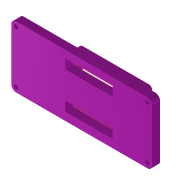
# Autodesk Inventor part: ESP32ParasiteMicroscope_base_v0
Saved by Autodesk Inventor 2022 (Build 260153000, 153)
## iProperties
Created: 2022-02-02
Part Number: ESP32ParasiteMicroscope_base_v0
Material: Generisch
Document SubType Name: Modeling
Designer: diederichbenedict
Density: 1 g/cm^3
Appearance: Glatt - Violett
Author: diederichbenedict
Autodesk Inventor part; units mm, degrees
ref_plane "YZ Plane" through (0, 0, 0) normal (1, 0, 0) x (0, 1, 0)
ref_plane "XZ Plane" through (0, 0, 0) normal (0, 1, 0) x (-1, 0, 0)
ref_plane "XY Plane" through (0, 0, 0) normal (0, 0, 1) x (1, 0, 0)
ref_plane "Arbeitsebene1" through (0, 0, 4) normal (0, 0, 1) x (1, 0, 0)
sketch "Skizze1" plane through (0, 0, 4) normal (0, 0, 1) x (1, 0, 0)
  arc A0 (-20, -12.5) -> (-19, -13.5) centre (-19, -12.5) ccw construction
  line L0 (-19, -13.5) -> (19, -13.5) construction
  arc A1 (19, -13.5) -> (20, -12.5) centre (19, -12.5) ccw construction
  line L1 (20, -12.5) -> (20, 12.5) construction
  arc A2 (20, 12.5) -> (19, 13.5) centre (19, 12.5) ccw construction
  line L2 (19, 13.5) -> (-19, 13.5) construction
  arc A3 (-19, 13.5) -> (-20, 12.5) centre (-19, 12.5) ccw construction
  line L3 (-20, 12.5) -> (-20, -12.5) construction
  line L4 (26, 12.5) -> (26, -12.5) construction
  arc A4 (19, -19.5) -> (26, -12.5) centre (19, -12.5) ccw construction
  line L5 (19, -19.5) -> (-19, -19.5) construction
  arc A5 (-26, -12.5) -> (-19, -19.5) centre (-19, -12.5) ccw construction
  line L6 (-26, -12.5) -> (-26, 12.5) construction
  arc A6 (-19, 19.5) -> (-26, 12.5) centre (-19, 12.5) ccw construction
  line L7 (-19, 19.5) -> (19, 19.5) construction
  arc A7 (26, 12.5) -> (19, 19.5) centre (19, 12.5) ccw construction
  line L8 (-24, 19.5) -> (19, 19.5)
  line L9 (19, 19.5) -> (19, -19.4749)
  line L10 (19, -19.4749) -> (-24, -19.4749)
  line L11 (-24, -19.4749) -> (-24, 19.5)
  line L12 (2.5735, 11.7657) -> (-15.3535, 11.7657) construction
  line L13 (2.5735, 13.7657) -> (-15.3535, 13.7657)
  line L14 (-15.3535, 9.7657) -> (2.5735, 9.7657)
  arc A8 (2.5735, 9.7657) -> (2.5735, 13.7657) centre (2.5735, 11.7657) ccw
  arc A9 (-15.3535, 13.7657) -> (-15.3535, 9.7657) centre (-15.3535, 11.7657) ccw
  line L15 (2.4395, -11.3613) -> (-15.3535, -11.3613) construction
  line L16 (2.4395, -9.3613) -> (-15.3535, -9.3613)
  line L17 (-15.3535, -13.3613) -> (2.4395, -13.3613)
  arc A10 (2.4395, -13.3613) -> (2.4395, -9.3613) centre (2.4395, -11.3613) ccw
  arc A11 (-15.3535, -9.3613) -> (-15.3535, -13.3613) centre (-15.3535, -11.3613) ccw
  circle A12 centre (-8.6034, 0.0126) radius 1.0539 construction
  line L18 (26.7026, 12.7126) -> (26.7026, -12.6874) construction
  line L19 (-48.7974, 12.7126) -> (26.7026, 12.7126) construction
  line L20 (-48.7974, -12.6874) -> (-48.7974, 12.7126) construction
  line L21 (26.7026, -12.6874) -> (-48.7974, -12.6874) construction
  line L22 (33.4901, -16.4749) -> (33.4901, 19.5) construction
  line L23 (30.4901, 19.5) -> (-52.5848, 19.5) construction
  line L24 (-55.5848, 19.5) -> (-55.5848, -16.4749) construction
  line L25 (-52.5848, -19.4749) -> (33.4901, -19.4749) construction
  line L26 (33.4901, 19.5) -> (19, 19.5)
  line L27 (19, 19.5) -> (19, -19.4749)
  line L28 (19, -19.4749) -> (30.4901, -19.4749)
  line L29 (33.4901, -19.4749) -> (33.4901, 16.5)
  line L30 (-24, 19.5) -> (-55.5848, 19.5)
  line L31 (-55.5848, 16.5) -> (-55.5848, -19.4749)
  line L32 (-55.5848, -19.4749) -> (-24, -19.4749)
  line L33 (-24, -19.4749) -> (-24, 19.5)
  arc A13 (-55.5848, -16.4749) -> (-52.5848, -19.4749) centre (-52.5848, -16.4749) ccw
  arc A14 (-52.5848, 19.5) -> (-55.5848, 16.5) centre (-52.5848, 16.5) ccw
  arc A15 (33.4901, 16.5) -> (30.4901, 19.5) centre (30.4901, 16.5) ccw
  arc A16 (30.4901, -19.4749) -> (33.4901, -16.4749) centre (30.4901, -16.4749) ccw
  line L34 (8.61, 8.7657) -> (-21.39, 8.7657)
  line L35 (-21.39, 8.7657) -> (-21.39, 14.7657)
  line L36 (-21.39, 14.7657) -> (8.61, 14.7657)
  line L37 (8.61, 14.7657) -> (8.61, 8.7657)
  line L38 (8.61, 8.7657) -> (-21.39, 14.7657) construction
  line L39 (-21.39, 8.7657) -> (8.61, 14.7657) construction
  line L40 (8.543, -14.3613) -> (-21.457, -14.3613)
  line L41 (-21.457, -14.3613) -> (-21.457, -8.3613)
  line L42 (-21.457, -8.3613) -> (8.543, -8.3613)
  line L43 (8.543, -8.3613) -> (8.543, -14.3613)
  line L44 (8.543, -14.3613) -> (-21.457, -8.3613) construction
  line L45 (-21.457, -14.3613) -> (8.543, -8.3613) construction
  point P0 (0, 0)
  point P1 (-15.2165, -11.3613)
  point P2 (-6.39, 11.7657)
  point P3 (-6.457, -11.3613)
  point P4 (-24, -18.4749)
  point P5 (33.4901, -16.4749)
  point P6 (30.4901, 19.5)
  point P7 (-52.5848, 19.5)
  point P8 (-55.5848, -16.4749)
  point P9 (-52.5848, -19.4749)
  dimension "d0" = 6
  dimension "d1" = 4
  dimension "d2" = 4
  dimension "d5" = 3
  dimension "d37" = 30
  dimension "d38" = 6
  dimension "d39" = 6
  dimension "d40" = 30
  constraints: 80 end point, 24 point on circle, 16 tangent, 15 parallel, 12 centre point, 9 point on line, 6 midpoint, 5 perpendicular, 4 horizontal, 3 equal radius, 14 other
  measures "d0" distance between parallel lines of L1 L4
  measures "d1" diameter of A9
  measures "d2" diameter of A11
  measures "d5" radius of A13
  measures "d37" distance of L34.start L34.end
  measures "d38" distance of L34.end L35.end
  measures "d39" distance of L40.end L41.end
  measures "d40" distance between parallel lines of L41 L43
extrude "Extrusion1" add sketch "Skizze1" along normal blind 5 contours L8 L9 L10 L11 | L11 L32 A13 L31 A14 L30 | L26 A15 L29 A16 L28 L9
sketch "Skizze3" plane through (0, 0, 4) normal (0, 0, -1) x (-1, 0, 0)
  arc A0 (-33.4901, -16.4749) -> (-30.4901, -19.4749) centre (-30.4901, -16.4749) ccw projected
  line L0 (52.5848, -19.4749) -> (-30.4901, -19.4749) projected
  arc A1 (52.5848, -19.4749) -> (55.5848, -16.4749) centre (52.5848, -16.4749) ccw projected
  line L1 (55.5848, 16.5) -> (55.5848, -16.4749) projected
  arc A2 (55.5848, 16.5) -> (52.5848, 19.5) centre (52.5848, 16.5) ccw projected
  line L2 (-30.4901, 19.5) -> (52.5848, 19.5) projected
  arc A3 (-30.4901, 19.5) -> (-33.4901, 16.5) centre (-30.4901, 16.5) ccw projected
  line L3 (-33.4901, -16.4749) -> (-33.4901, 16.5) projected
  circle A4 centre (-30.4901, 16.5) radius 1.15
  circle A5 centre (-30.4901, -16.4749) radius 1.4
  circle A6 centre (52.5848, 16.5) radius 1.4
  circle A7 centre (52.5848, -16.4749) radius 1.4
  point P0 (0, 0)
  dimension "d16" = 2.3
  dimension "d17" = 2.8
  dimension "d18" = 2.8
  dimension "d19" = 2.8
  constraints: 4 centre point, 4 coincident
  measures "d16" diameter of A4
  measures "d17" diameter of A5
  measures "d18" diameter of A6
  measures "d19" diameter of A7
extrude "Extrusion3" cut sketch "Skizze3" against normal blind 10 contours A4 | A5 | A6 | A7
ref_plane "Arbeitsebene2" through (20, 13.5, 0) normal (1, 0, 0) x (0, 0, -1)
ref_plane "Arbeitsebene3" through (-20, -12.5, -1) normal (-1, 0, 0) x (0, 0, 1)
sketch "Skizze4" plane through (20, 13.5, 0) normal (1, 0, 0) x (0, 0, -1)
  line L0 (0, -27) -> (1, -27)
  line L1 (0, -27) -> (0, -26)
  line L2 (1, -26) -> (1, -27)
  line L3 (1, 0) -> (1, -1)
  line L4 (1, 0) -> (0, 0)
  line L5 (0, -1) -> (0, 0)
  line L6 (-4, -29.9749) -> (-4, 3)
  line L7 (-4, -0.3) -> (0, -0.3)
  line L8 (0, -0.3) -> (0, 3)
  line L9 (0, 3) -> (-4, 3)
  line L10 (-4, 3) -> (-4, -0.3)
  line L11 (0, -26.5) -> (-4, -26.5)
  line L12 (-4, -26.5) -> (-4, -30)
  line L13 (-4, -30) -> (0, -30)
  line L14 (0, -30) -> (0, -26.5)
  line L15 (0, 3) -> (1.5, 3)
  line L16 (1.5, 3) -> (1.5, 0.25)
  line L17 (1.5, 0.25) -> (0, 0.25)
  line L18 (0, 0.25) -> (0, 3)
  line L19 (0, -30) -> (1.5, -30)
  line L20 (1.5, -30) -> (1.5, -27.25)
  line L21 (1.5, -27.25) -> (0, -27.25)
  line L22 (0, -27.25) -> (0, -30)
  line L23 (1, 0) -> (0, 0)
  point P0 (0, -13.5)
  point P1 (0, -27.25)
  point P2 (-4, 3)
  point P3 (0, -0.3)
  point P4 (0, 0.25)
extrude "Extrusion4" add sketch "Skizze4" against normal up to surface (40 mm away)
sketch "Skizze5" plane through (20, 16.5, 4) normal (0, 1, 0) x (1, 0, 0)
  line L0 (-40, 4) -> (-40, 5) projected
  line L1 (0, 5) -> (0, 4) projected
  line L2 (0, 5.5) -> (-40, 5.5) projected
  line L3 (-40, 5.5) -> (-40, 0) projected
  line L4 (0, 4) -> (-40, 4) projected
  line L5 (-40, 0) -> (-43, 0)
  line L6 (-43, 0) -> (-43, 4)
  line L7 (-43, 4) -> (-40, 4)
  line L8 (-40, 4) -> (-40, 0)
  line L9 (-43, 4) -> (-41, 4)
  line L10 (-41, 4) -> (-41, 5.5)
  line L11 (-41, 5.5) -> (-43, 5.5)
  line L12 (-43, 5.5) -> (-43, 4)
  line L13 (0, 5.5) -> (0, 0) projected
  line L14 (0, 0) -> (3, 0)
  line L15 (3, 0) -> (3, 4)
  line L16 (3, 4) -> (0, 4)
  line L17 (0, 4) -> (0, 0)
  line L18 (3, 4) -> (1, 4)
  line L19 (1, 4) -> (1, 5.5)
  line L20 (1, 5.5) -> (3, 5.5)
  line L21 (3, 5.5) -> (3, 4)
  point P0 (-20, 4)
  point P1 (1, 4)
  point P2 (0, 4)
  dimension "d31" = 3
  dimension "d32" = 2
  dimension "d33" = 3
  dimension "d34" = 2
  constraints: 32 end point, 8 parallel, 4 horizontal, 4 perpendicular
  measures "d31" distance of L6.end L7.end
  measures "d32" distance of L11.end L10.end
  measures "d33" distance of L16.end L15.end
  measures "d34" distance of L19.end L20.end
extrude "Extrusion5" add sketch "Skizze5" against normal up to surface (33 mm away) contours L16 L15 L14 L13 | L3 L5 L6 L7 | L7 L12 L11 L10 | L19 L20 L21 L16
sketch "Skizze6" plane through (23, 16.5, -1.5) normal (0, 0, -1) x (-1, 0, 0)
  line L0 (0, -33) -> (2, -33) projected
  line L1 (2, 0) -> (2, -33) projected
  line L2 (0, 0) -> (2, 0) projected
  line L3 (0, 0) -> (0, -33) projected
  line L4 (44, -33) -> (46, -33) projected
  line L5 (46, 0) -> (46, -33) projected
  line L6 (44, 0) -> (46, 0) projected
  line L7 (44, 0) -> (44, -33) projected
  line L8 (3, -30.25) -> (43, -30.25) projected
  line L9 (3, -2.75) -> (43, -2.75) projected
  line L10 (0, 0) -> (0, -33) projected
  line L11 (0, 0) -> (46, 0)
  line L12 (46, 0) -> (46, -33)
  line L13 (46, -33) -> (0, -33)
  line L14 (0, -33) -> (0, 0)
  line L15 (2, 0) -> (2, -33) projected
  line L16 (2, -2.75) -> (44, -2.75)
  line L17 (44, -2.75) -> (44, -30.25)
  line L18 (44, -30.25) -> (2, -30.25)
  line L19 (2, -30.25) -> (2, -2.75)
  point P0 (23, -16.5)
  point P1 (44, -2.75)
  point P2 (2, -30.25)
  constraints: 16 end point, 4 parallel, 2 horizontal, 2 perpendicular, 2 point on line
extrude "Extrusion6" add sketch "Skizze6" against normal up to surface (1.5 mm away) contours L3 L2 L1 L0 | L1 L18 L8 L7 L13 | L7 L6 L5 L4 | L11 L7 L16 L9 L1
fillet "Rundung1" radius 2 9 edges at (23, -16.5, 1.25) (-23, -16.5, 1.25) (-23, 16.5, 1.25) (23, 16.5, 1.25) (21, 13.75, -0.75) (20, 13.2, 2) (21, -13.75, -0.75) (-21, -13.75, -0.75) (-21, 13.75, -0.75)
sketch "Skizze7" plane through (21, 16.5, -1.5) normal (0, 0, -1) x (-1, 0, 0)
  point P0 (21, -16.5)
sketch "Skizze8" plane through (21, 16.5, -1.5) normal (0, 0, -1) x (-1, 0, 0)
  line L0 (40, -30.25) -> (2, -30.25) projected
  arc A0 (0, -28.25) -> (2, -30.25) centre (2, -28.25) ccw projected
  line L1 (0, -4.75) -> (0, -28.25) projected
  arc A1 (2, -2.75) -> (0, -4.75) centre (2, -4.75) ccw projected
  line L2 (2, -2.75) -> (40, -2.75) projected
  arc A2 (42, -4.75) -> (40, -2.75) centre (40, -4.75) ccw projected
  line L3 (42, -4.75) -> (42, -28.25) projected
  arc A3 (40, -30.25) -> (42, -28.25) centre (40, -28.25) ccw projected
  arc A4 (0, 0) -> (-2, -2) centre (0, -2) ccw projected
  line L4 (-2, -2) -> (-2, -31) projected
  arc A5 (-2, -31) -> (0, -33) centre (0, -31) ccw projected
  line L5 (0, -33) -> (42, -33) projected
  arc A6 (42, -33) -> (44, -31) centre (42, -31) ccw projected
  line L6 (44, -2) -> (44, -31) projected
  arc A7 (44, -2) -> (42, 0) centre (42, -2) ccw projected
  line L7 (0, 0) -> (42, 0) projected
  point P0 (21, -16.5)
extrude "Extrusion7" cut sketch "Skizze8" against normal blind 3 contours L0 A0 L1 A1 L2 A2 L3 A3
